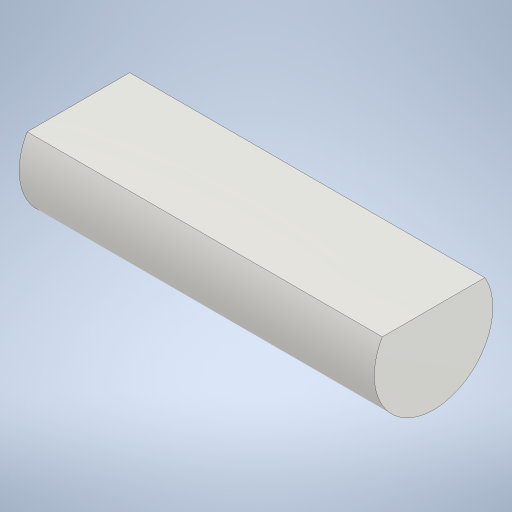
# Autodesk Inventor part: Shaft
Saved by Autodesk Inventor 2023 (Build 270158000, 158)
## iProperties
CustomPartVersion: 1
Created: 2023-05-29
Part Number: Shaft
Material: Steel
Document SubType Name: Modeling
Designer: Ronan
Density: 1 g/cm^3
Appearance: Steel
Length: 18,000 mm
Author: Ronan
Autodesk Inventor part; units mm, degrees
ref_plane "Start Plane" through (0, 0, 0) normal (1, 0, 0) x (0, 1, 0)
ref_plane "XZ Plane" through (0, 0, 0) normal (0, 1, 0) x (-1, 0, 0)
ref_plane "XY Plane" through (0, 0, 0) normal (0, 0, 1) x (1, 0, 0)
sketch "Main Sketch" plane through (0, 0, 0) normal (0, 0, 1) x (1, 0, 0)
  line L0 (0, 0) -> (18, 0)
  line L1 (0, 0) -> (0, 3)
  line L2 (18, 3) -> (18, 0)
  line L3 (0, 3) -> (18, 3)
  dimension "d3" = 6
  constraints: 8 end point, 3 horizontal, 2 vertical
  measures "d3" diameter of L3 L0
revolve "Revolution1" add sketch "Main Sketch" angle 360 about axis through (0, 0, 0) along (1, 0, 0)
sketch "Sketch3" plane through (0, 0, 0) normal (-1, 0, 0) x (0, 0, 1)
  circle A0 centre (0, 0) radius 3 projected
  line L0 (-2.5981, 1.5) -> (2.5981, 1.5)
  circle A1 centre (0, 0) radius 3
  dimension "d8" = 1.5
  constraints: 2 end point, 2 point on circle, 1 centre point, 1 coincident, 1 concentric, 1 horizontal
  measures "d8" distance from line of point (0, 0) L0
extrude "Extrusion1" cut sketch "Sketch3" against normal through all contours L0 A0 picked at (0.7274, 1.6862)
equation "\"Length\" = 18"
body "Solid1"
